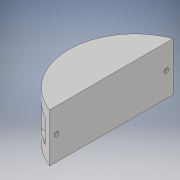
# Autodesk Inventor part: joint3_cap
Saved by Autodesk Inventor 2019 (Build 230136000, 136)
## iProperties
Created: 2019-12-29
Part Number: joint3_cap
Material: Типовые
Document SubType Name: Modeling
Designer: Петров Иван
Density: 1 g/cm^3
Appearance: По умолчанию
Author: Петров Иван
Autodesk Inventor part; units mm, degrees
ref_plane "YZ Plane" through (0, 0, 0) normal (1, 0, 0) x (0, 1, 0)
ref_plane "XZ Plane" through (0, 0, 0) normal (0, 1, 0) x (-1, 0, 0)
sketch "Эскиз1" plane through (0, 0, 0) normal (0, 1, 0) x (-1, 0, 0)
  circle A0 centre (0, 0) radius 3.9
  line L0 (-35, -37.5) -> (-35, 37.5)
  line L1 (-35, -37.5) -> (15, -37.5)
  line L2 (15, -37.5) -> (15, -39.7649)
  arc A1 (15, -39.7649) -> (15, 39.7649) centre (0, 0) ccw
  line L3 (15, 39.7649) -> (15, 37.5)
  line L4 (-35, 37.5) -> (15, 37.5)
  line L5 (15, 39.7649) -> (15, -39.7649)
  point P0 (-39, 0)
  constraints: 12 end point, 2 centre point, 2 point on circle, 1 vertical
extrude "Выдавливание1" add sketch "Эскиз1" along normal blind 31.32 contours L5 L3 A1 L2
ref_plane "РабПлоскость1" through (-42.5, 0, 0) normal (1, 0, 0) x (0, 1, 0)
sketch "Эскиз2" plane through (-42.5, 0, 0) normal (1, 0, 0) x (0, 1, 0)
  line L0 (31.32, -39.7649) -> (31.32, 39.7649) projected
  line L1 (31.32, -39.7649) -> (15.66, -39.7649)
  line L2 (0, -39.7649) -> (31.32, -39.7649) projected
  line L3 (15.66, -39.7649) -> (15.66, -34.7649)
  line L4 (8.16, -39.7649) -> (23.16, -39.7649)
  line L5 (23.16, -39.7649) -> (23.16, -29.7649)
  line L6 (23.16, -29.7649) -> (8.16, -29.7649)
  line L7 (8.16, -29.7649) -> (8.16, -39.7649)
  line L8 (8.16, -39.7649) -> (23.16, -29.7649) construction
  line L9 (23.16, -39.7649) -> (8.16, -29.7649) construction
  line L10 (31.32, 0) -> (24.2001, 0)
  line L11 (31.32, 39.7649) -> (15.66, 39.7649)
  line L12 (0, 39.7649) -> (31.32, 39.7649)
  line L13 (15.66, 39.7649) -> (15.66, 34.7649)
  line L14 (8.16, 39.7649) -> (23.16, 39.7649)
  line L15 (23.16, 39.7649) -> (23.16, 29.7649)
  line L16 (23.16, 29.7649) -> (8.16, 29.7649)
  line L17 (8.16, 29.7649) -> (8.16, 39.7649)
  line L18 (8.16, 39.7649) -> (23.16, 29.7649) construction
  line L19 (23.16, 39.7649) -> (8.16, 29.7649) construction
  point P0 (0, 0)
  dimension "d2" = 15.66
  dimension "d3" = 5
  dimension "d4" = 15
  dimension "d5" = 10
  constraints: 36 end point, 7 symmetric about line, 6 midpoint, 2 horizontal, 2 parallel, 2 perpendicular
  measures "d2" distance of L0.start L1.end
  measures "d3" distance of L1.end L3.end
  measures "d4" distance of L6.end L5.end
  measures "d5" distance of L5.end L4.end
extrude "Выдавливание2" cut sketch "Эскиз2" along normal blind 22.32
sketch "Эскиз3" plane through (-42.5, 0, 0) normal (1, 0, 0) x (0, 1, 0)
  line L0 (8.16, -37.4034) -> (23.16, -37.4034) projected
  line L1 (15.66, -37.4034) -> (15.66, -35.4034)
  circle A0 centre (15.66, -35.4034) radius 1.5
  line L2 (23.16, 37.4034) -> (8.16, 37.4034) projected
  line L3 (15.66, 37.4034) -> (15.66, 35.4034)
  circle A1 centre (15.66, 35.4034) radius 1.5
  point P0 (0, 0)
  dimension "d8" = 2
  dimension "d9" = 3
  dimension "d10" = 2
  dimension "d11" = 3
  constraints: 4 end point, 2 centre point, 2 coincident, 2 midpoint, 2 vertical
  measures "d8" distance of L1.start L1.end
  measures "d9" diameter of A0
  measures "d10" distance of L3.start L3.end
  measures "d11" diameter of A1
extrude "Выдавливание3" cut sketch "Эскиз3" along normal through all
